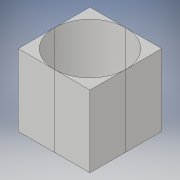
# Autodesk Inventor part: gdhole
Saved by Autodesk Inventor 2017 (Build 210142000, 142)
## iProperties
Created: 2016-10-12
Part Number: gdhole
Material: Generic
Document SubType Name: Modeling
Designer: Aditya
Density: 1 g/cm^3
Appearance: Default
Author: Aditya
Autodesk Inventor part; units mm, degrees
ref_plane "YZ Plane" through (0, 0, 0) normal (1, 0, 0) x (0, 1, 0)
ref_plane "XZ Plane" through (0, 0, 0) normal (0, 1, 0) x (-1, 0, 0)
ref_plane "XY Plane" through (0, 0, 0) normal (0, 0, 1) x (1, 0, 0)
sketch "Sketch1" plane through (0, 0, 0) normal (0, 1, 0) x (-1, 0, 0)
  line L0 (0, 0) -> (0, -1752.6)
  line L1 (0, -1752.6) -> (1752.6, -1752.6)
  line L2 (1752.6, -1752.6) -> (1752.6, 0)
  line L3 (1752.6, 0) -> (0, 0)
  circle A0 centre (876.3, -876.3) radius 876.3
  dimension "d0" = 1752.6
  dimension "d1" = 1752.6
  constraints: 8 end point, 3 perpendicular, 1 centre point, 1 tangent, 1 vertical
  measures "d0" distance of L0.start L0.end
  measures "d1" distance of L0.end L1.end
extrude "Extrusion1" add sketch "Sketch1" along normal blind 1752.6 contours L3 A0 L0 | A0 L1 L0 | L3 L2 A0 | A0 L2 L1
body "Solid1"
